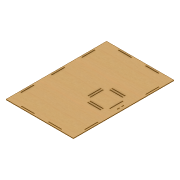
# Autodesk Inventor part: основание
Saved by Autodesk Inventor 2021 (Build 250183000, 183)
## iProperties
Created: 2023-02-14
Part Number: основание
Material: Типовые
Document SubType Name: Modeling
Designer: Tasya
Density: 1 g/cm^3
Appearance: Желтая сосна — массив — светлое морение — со слабым глянцем
Author: Tasya
Autodesk Inventor part; units mm, degrees
ref_plane "YZ Plane" through (0, 0, 0) normal (1, 0, 0) x (0, 1, 0)
ref_plane "XZ Plane" through (0, 0, 0) normal (0, 1, 0) x (-1, 0, 0)
ref_plane "XY Plane" through (0, 0, 0) normal (0, 0, 1) x (1, 0, 0)
sketch "Эскиз1" plane through (0, 0, 0) normal (0, 1, 0) x (-1, 0, 0)
  line L0 (-225, 340.5) -> (225, 340.5) construction
  line L1 (225, 340.5) -> (225, -340.5) construction
  line L2 (225, -340.5) -> (-225, -340.5) construction
  line L3 (-225, -340.5) -> (-225, 340.5) construction
  line L4 (-225, 340.5) -> (225, -340.5) construction
  line L5 (225, 340.5) -> (-225, -340.5) construction
  line L6 (-185, -70.5) -> (-45, -70.5) construction
  line L7 (-45, -70.5) -> (-45, 70.5) construction
  line L8 (-45, 70.5) -> (-185, 70.5) construction
  line L9 (-185, 70.5) -> (-185, -70.5) construction
  line L10 (-185, -70.5) -> (-45, 70.5) construction
  line L11 (-45, -70.5) -> (-185, 70.5) construction
  line L12 (221, -336.5) -> (221, 336.5) construction
  line L13 (221, 336.5) -> (-221, 336.5) construction
  line L14 (-221, -336.5) -> (221, -336.5) construction
  line L15 (263.1324, 0) -> (0, 0) construction
  line L16 (-221, 86.5) -> (-29, 86.5) construction
  line L17 (-29, 86.5) -> (-29, -86.5) construction
  line L18 (-29, -86.5) -> (-221, -86.5) construction
  line L19 (-225, 82.5) -> (-33, 82.5) construction
  line L20 (-33, 82.5) -> (-33, -82.5) construction
  line L21 (-33, -82.5) -> (-225, -82.5) construction
  line L22 (-221, 336.5) -> (-221, 86.5) construction
  line L23 (-221, -86.5) -> (-221, -336.5) construction
  line L24 (-95.3724, 0) -> (-115, 0) construction
  line L25 (-115, 0) -> (-115, -31.3675) construction
  line L26 (-70, 70.5) -> (-160, 70.5)
  line L27 (-160, 70.5) -> (-160, 66.5)
  line L28 (-160, 66.5) -> (-70, 66.5)
  line L29 (-70, 66.5) -> (-70, 70.5)
  line L30 (-181.5, -45) -> (-181.5, 45)
  line L31 (-181.5, 45) -> (-185.5, 45)
  line L32 (-185.5, -45) -> (-181.5, -45)
  line L33 (-185.5, 45) -> (-185.5, -45)
  line L34 (-70, -66.5) -> (-160, -66.5)
  line L35 (-160, -66.5) -> (-160, -70.5)
  line L36 (-70, -70.5) -> (-70, -66.5)
  line L37 (-160, -70.5) -> (-70, -70.5)
  line L38 (-48.5, 45) -> (-48.5, -45)
  line L39 (-48.5, -45) -> (-44.5, -45)
  line L40 (-44.5, 45) -> (-48.5, 45)
  line L41 (-44.5, -45) -> (-44.5, 45)
  line L42 (235, 350.5) -> (-235, 350.5)
  line L43 (-235, 350.5) -> (-235, -350.5)
  line L44 (-235, -350.5) -> (235, -350.5)
  line L45 (235, -350.5) -> (235, 350.5)
  line L46 (140, 340.5) -> (50, 340.5)
  line L47 (50, 340.5) -> (50, 336.5)
  line L48 (50, 336.5) -> (140, 336.5)
  line L49 (140, 336.5) -> (140, 340.5)
  line L50 (-50, 340.5) -> (-140, 340.5)
  line L51 (-140, 340.5) -> (-140, 336.5)
  line L52 (-140, 336.5) -> (-50, 336.5)
  line L53 (-50, 336.5) -> (-50, 340.5)
  line L54 (0, 0) -> (0, -86) construction
  line L55 (140, -340.5) -> (50, -340.5)
  line L56 (50, -340.5) -> (50, -336.5)
  line L57 (50, -336.5) -> (140, -336.5)
  line L58 (140, -336.5) -> (140, -340.5)
  line L59 (-50, -340.5) -> (-140, -340.5)
  line L60 (-140, -340.5) -> (-140, -336.5)
  line L61 (-140, -336.5) -> (-50, -336.5)
  line L62 (-50, -336.5) -> (-50, -340.5)
  line L63 (-225, 258.5) -> (-225, 168.5)
  line L64 (-225, 168.5) -> (-221, 168.5)
  line L65 (-221, 168.5) -> (-221, 258.5)
  line L66 (-221, 258.5) -> (-225, 258.5)
  line L67 (-225, -166.5) -> (-225, -256.5)
  line L68 (-225, -256.5) -> (-221, -256.5)
  line L69 (-221, -256.5) -> (-221, -166.5)
  line L70 (-221, -166.5) -> (-225, -166.5)
  line L71 (-29, 45) -> (-29, -45)
  line L72 (-29, -45) -> (-33, -45)
  line L73 (-33, -45) -> (-33, 45)
  line L74 (-33, 45) -> (-29, 45)
  line L75 (-70, -82.5) -> (-70, -86.5)
  line L76 (-70, -86.5) -> (-160, -86.5)
  line L77 (-160, -86.5) -> (-160, -82.5)
  line L78 (-160, -82.5) -> (-70, -82.5)
  line L79 (-70, 82.5) -> (-70, 86.5)
  line L80 (-70, 86.5) -> (-160, 86.5)
  line L81 (-160, 86.5) -> (-160, 82.5)
  line L82 (-160, 82.5) -> (-70, 82.5)
  line L83 (225, 258.5) -> (225, 168.5)
  line L84 (225, 168.5) -> (221, 168.5)
  line L85 (221, 168.5) -> (221, 258.5)
  line L86 (221, 258.5) -> (225, 258.5)
  line L87 (221, 45) -> (221, -45)
  line L88 (221, -45) -> (225, -45)
  line L89 (225, -45) -> (225, 45)
  line L90 (225, 45) -> (221, 45)
  line L91 (221, -166.5) -> (221, -256.5)
  line L92 (221, -256.5) -> (225, -256.5)
  line L93 (225, -256.5) -> (225, -166.5)
  line L94 (225, -166.5) -> (221, -166.5)
  line L95 (-235, -72.3208) -> (-235, 372.16)
  line L96 (-215, 22.5) -> (-211, 22.5)
  line L97 (-211, 22.5) -> (-211, 7.5)
  line L98 (-211, 7.5) -> (-215, 7.5)
  line L99 (-215, 7.5) -> (-215, 22.5)
  line L100 (-215, -7.5) -> (-211, -7.5)
  line L101 (-211, -7.5) -> (-211, -22.5)
  line L102 (-211, -22.5) -> (-215, -22.5)
  line L103 (-215, -22.5) -> (-215, -7.5)
  circle A0 centre (-213, 0) radius 2.6 construction
  line L104 (-213, -7.5) -> (-213, 7.5) construction
  point P0 (-213, -22.5)
  dimension "d13" = 140
  dimension "d14" = 141
  dimension "d15" = 4
  dimension "d17" = 16
  dimension "d18" = 16
  dimension "d19" = 16
  dimension "d20" = 4
  dimension "d22" = 4
  dimension "d23" = 4
  dimension "d24" = 250
  dimension "d25" = 4
  dimension "d26" = 4
  dimension "d27" = 250
  dimension "d28" = 90
  dimension "d29" = 4
  dimension "d32" = 360
  dimension "d34" = 4
  dimension "d35" = 10
  dimension "d36" = 50
  dimension "d37" = 90
  dimension "d39" = 100
  dimension "d40" = 90
  dimension "d41" = 86
  dimension "d42" = 84
  dimension "d56" = 4
  dimension "d57" = 4
  dimension "d58" = 15
  dimension "d59" = 20
  dimension "d62" = 5.2
  dimension "d70" = 15
  constraints: 210 end point, 34 point on line, 26 parallel, 18 perpendicular, 13 collinear, 8 midpoint, 8 symmetric about line, 6 equal length, 6 horizontal, 5 vertical, 1 centre point, 1 horizontal alignment, 40 other
  measures "d13" distance of L7.end L8.end
  measures "d14" distance of L6.end L7.end
  measures "d15" distance between parallel lines of L1 L12
  measures "d17" distance between parallel lines of L6 L18
  measures "d18" distance between parallel lines of L7 L17
  measures "d19" distance between parallel lines of L16 L8
  measures "d20" distance between parallel lines of L17 L20
  measures "d22" distance between parallel lines of L16 L19
  measures "d23" distance between parallel lines of L18 L21
  measures "d24" distance between parallel lines of L17 L12
  measures "d25" distance between parallel lines of L3 L22
  measures "d26" distance between parallel lines of L2 L14
  measures "d27" distance between parallel lines of L16 L13
  measures "d28" distance of L27.end L28.end
  measures "d29" distance of L26.end L27.end
  measures "d34" distance between parallel lines of L13 L0
  measures "d35" distance between parallel lines of L0 L42
  measures "d36" distance between parallel lines of L43 L9
  measures "d37" distance of L47.end L48.end
  measures "d39" distance from line of L50.start L47
  measures "d40" distance of L84.end L85.end
  measures "d41" distance between parallel lines of L19 L64
  measures "d42" distance between parallel lines of L21 L70
  measures "d56" distance of L101.end L103.start
  measures "d57" distance of L99.end L97.start
  measures "d58" distance between parallel lines of L98 L100
  measures "d59" distance between parallel lines of L95 L103
  measures "d62" diameter of A0
  measures "d70" distance between parallel lines of L98 L96
extrude "Выдавливание1" add sketch "Эскиз1" along normal blind 4
sketch "Эскиз3" plane through (0, 0, 0) normal (0, 1, 0) x (1, 0, 0)
  circle A0 centre (213, 0) radius 2.6 construction
  point P0 (0, 0)
hole "Отверстие1" at (213, 0, 0) direction (0, 1, 0) diameter 5.2 depth 1.7
equation "\"d18\" = d17"
equation "\"d19\" = d17"
equation "\"d20\" = d15"
equation "\"d22\" = d20"
equation "\"d23\" = d20"
equation "\"d25\" = d34"
equation "\"d26\" = d15"
equation "\"d28\" = d40"
equation "\"d29\" = d15"
equation "\"d34\" = d15"
equation "\"d37\" = d40"
